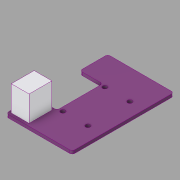
# Autodesk Inventor part: Sensor Board
Saved by Autodesk Inventor 2017 (Build 210142000, 142)
## iProperties
Created: 2017-02-20
Part Number: Sensor Board
Material: Generic
Document SubType Name: Modeling
Designer: qupec
Density: 1 g/cm^3
Appearance: Default
Author: qupec
Autodesk Inventor part; units mm, degrees
ref_plane "YZ Plane" through (0, 0, 0) normal (1, 0, 0) x (0, 1, 0)
ref_plane "XZ Plane" through (0, 0, 0) normal (0, 1, 0) x (-1, 0, 0)
ref_plane "XY Plane" through (0, 0, 0) normal (0, 0, 1) x (1, 0, 0)
sketch "Sketch1" plane through (0, 0, 0) normal (0, 1, 0) x (-1, 0, 0)
  line L0 (16.51, 25.4) -> (-16.51, 25.4)
  line L1 (-16.51, 25.4) -> (-16.51, -25.4)
  line L2 (-16.51, -25.4) -> (16.51, -25.4)
  line L3 (16.51, -25.4) -> (16.51, -11.43)
  line L4 (16.51, -11.43) -> (5.08, -11.43)
  line L5 (5.08, -11.43) -> (5.08, 11.43)
  line L6 (5.08, 11.43) -> (16.51, 11.43)
  line L7 (16.51, 11.43) -> (16.51, 25.4)
  point P0 (0, 0)
  dimension "d0" = 33.02
  dimension "d1" = 33.02
  dimension "d2" = 16.51
  dimension "d3" = 50.8
  dimension "d4" = 25.4
  dimension "d7" = 11.43
  dimension "d8" = 22.86
  dimension "d9" = 11.43
  constraints: 16 end point, 7 perpendicular, 1 horizontal
  measures "d0" distance between parallel lines of L1 L7
  measures "d1" distance between parallel lines of L1 L3
  measures "d2" distance from line of point (0, 0) L7
  measures "d3" distance between parallel lines of L2 L0
  measures "d4" distance from line of point (0, 0) L0
  measures "d7" distance between parallel lines of L7 L5
  measures "d8" distance between parallel lines of L4 L6
  measures "d9" distance from line of point (0, 0) L6
extrude "Extrusion1" add sketch "Sketch1" along normal blind 1.6
fillet "Fillet1" radius 1.27 8 edges at (16.51, 0.8, 25.4) (-16.51, 0.8, 25.4) (-16.51, 0.8, -25.4) (16.51, 0.8, -25.4) (-5.08, 0.8, -11.43) (-5.08, 0.8, 11.43) (-16.51, 0.8, -11.43) (-16.51, 0.8, 11.43)
sketch "Sketch2" plane through (0, 1.6, 0) normal (0, 1, 0) x (1, 0, 0)
  arc A0 (-16.51, -24.13) -> (-15.24, -25.4) centre (-15.24, -24.13) ccw projected
  line L0 (-15.24, -24.13) -> (-6.35, -24.13)
  line L1 (-6.35, -24.13) -> (-6.35, -12.7)
  line L2 (-6.35, -12.7) -> (-15.24, -12.7)
  line L3 (-15.24, -12.7) -> (-15.24, -24.13)
  line L4 (-15.24, -25.4) -> (15.24, -25.4) projected
  line L5 (-6.35, -11.43) -> (-15.24, -11.43) projected
  point P0 (0, 0)
  dimension "d13" = 11.43
  dimension "d14" = 1.27
  dimension "d15" = 1.27
  dimension "d16" = 8.89
  constraints: 8 end point, 2 parallel, 1 horizontal, 1 perpendicular
  measures "d13" distance between parallel lines of L2 L0
  measures "d14" distance between parallel lines of L4 L0
  measures "d15" distance between parallel lines of L5 L2
  measures "d16" distance between parallel lines of L1 L3
extrude "Extrusion2" add sketch "Sketch2" along normal blind 12.7
sketch "Sketch3" plane through (0, 1.6, 0) normal (0, 1, 0) x (1, 0, 0)
  circle A0 centre (-3.0683, -10.5016) radius 1.143
  circle A1 centre (-3.0683, 10.5016) radius 1.143
  circle A2 centre (9.431, -10.5016) radius 1.143
  circle A3 centre (9.431, 10.5016) radius 1.143
  line L0 (16.51, -24.13) -> (16.51, 24.13) projected
  point P0 (0, 0)
  dimension "d19" = 2.286
  dimension "d20" = 2.286
  dimension "d21" = 2.286
  dimension "d22" = 2.286
  dimension "d23" = 21.0033
  dimension "d24" = 21.0033
  dimension "d25" = 10.5016
  dimension "d26" = 10.5016
  dimension "d27" = 12.4993
  dimension "d28" = 7.079
  dimension "d29" = 7.079
  dimension "d30" = 12.4993
  constraints: 4 centre point
  measures "d19" diameter of A0
  measures "d20" diameter of A1
  measures "d21" diameter of A2
  measures "d22" diameter of A3
  measures "d23" distance of A3.centre A2.centre
  measures "d24" distance of A1.centre A0.centre
  measures "d25" vertical distance of point (0, 0) A2.centre
  measures "d26" vertical distance of point (0, 0) A0.centre
  measures "d27" distance of A2.centre A0.centre
  measures "d28" distance from line of L0 A2.centre
  measures "d29" distance from line of A3.centre L0
  measures "d30" distance of A3.centre A1.centre
extrude "Extrusion3" cut sketch "Sketch3" against normal through all
equation "\"d1\" = d0"
equation "\"d2\" = 0.5 * d0"
equation "\"d4\" = 0.5 * d3"
equation "\"d9\" = 0.5 * d8"
equation "\"d15\" = d14"
equation "\"d20\" = d19"
equation "\"d21\" = d20"
equation "\"d22\" = d21"
equation "\"d24\" = d23"
equation "\"d25\" = 0.5 * d23"
equation "\"d26\" = 0.5 * d24"
equation "\"d29\" = d28"
equation "\"d30\" = d27"
body "Solid1"
